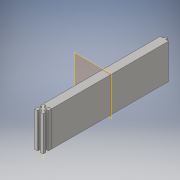
# Autodesk Inventor part: mazeblock
Saved by Autodesk Inventor 2016 (Build 200138000, 138)
## iProperties
Created: 2016-04-28
Part Number: mazeblock
Material: Generic
Document SubType Name: Modeling
Designer: brent
Density: 1 g/cm^3
Appearance: Default
Author: brent
Autodesk Inventor part; units mm, degrees
ref_plane "YZ Plane" through (0, 0, 0) normal (1, 0, 0) x (0, 1, 0)
ref_plane "XZ Plane" through (0, 0, 0) normal (0, 1, 0) x (-1, 0, 0)
ref_plane "XY Plane" through (0, 0, 0) normal (0, 0, 1) x (1, 0, 0)
sketch "Sketch1" plane through (0, 0, 0) normal (0, 1, 0) x (-1, 0, 0)
  line L0 (0, 0) -> (-180, 0) construction
  line L1 (-180, 0) -> (-180, -180) construction
  line L2 (-180, -180) -> (0, -180) construction
  line L3 (0, -180) -> (0, 0) construction
  line L4 (-6, 6) -> (6, 6)
  line L5 (6, 6) -> (6, -6)
  line L6 (6, -6) -> (1.2361, -6)
  line L7 (-6, -6) -> (-6, 6)
  line L8 (-6, 6) -> (6, -6) construction
  line L9 (6, 6) -> (-6, -6) construction
  line L10 (-6, -174) -> (6, -174)
  line L11 (6, -174) -> (6, -186)
  line L12 (6, -186) -> (-6, -186)
  line L13 (-6, -186) -> (-6, -174)
  line L14 (-6, -174) -> (6, -186) construction
  line L15 (6, -174) -> (-6, -186) construction
  line L16 (-6, -6.2) -> (6, -6.2)
  line L17 (6, -6.2) -> (6, -173.8)
  line L18 (6, -173.8) -> (-6, -173.8)
  line L19 (-6, -173.8) -> (-6, -6.2)
  line L20 (-6, -6.2) -> (6, -173.8) construction
  line L21 (6, -6.2) -> (-6, -173.8) construction
  line L22 (0, -2.1958) -> (2, -3.6489)
  line L23 (2, -3.6489) -> (1.2361, -6)
  line L24 (-1.2361, -6) -> (-2, -3.6489)
  line L25 (-2, -3.6489) -> (0, -2.1958)
  line L26 (0, -2.4739) -> (1.7355, -3.7348)
  line L27 (1.7355, -3.7348) -> (1.0726, -5.775)
  line L28 (-1.0726, -5.775) -> (-1.7355, -3.7348)
  line L29 (-1.7355, -3.7348) -> (0, -2.4739)
  line L30 (1.0726, -5.775) -> (0.9345, -6.2)
  line L31 (-1.0726, -5.775) -> (-0.9345, -6.2)
  line L32 (1.2361, -6) -> (-1.2361, -6)
  line L33 (-1.2361, -6) -> (-6, -6)
  line L34 (6, -6.2) -> (5, -6.2)
  line L35 (5, -6.2) -> (5, -6.15)
  line L36 (5, -6.15) -> (6, -6.15)
  line L37 (6, -6.15) -> (6, -6.2)
  line L38 (-5, -6.2) -> (-5, -6.15)
  line L39 (-5, -6.15) -> (-6, -6.15)
  line L40 (-6, -6.15) -> (-6, -6.2)
  line L41 (5, -6.2) -> (6, -6.2)
  line L42 (-6, -6.2) -> (-5, -6.2)
  point P0 (0, -90)
  point P1 (0, -4.2987)
  point P2 (0, -4.2987)
  dimension "d0" = 180
  dimension "d1" = 180
  dimension "d4" = 12
  dimension "d5" = 12
  dimension "d6" = 0.2
  dimension "d7" = 4
  dimension "d8" = 0.225
  dimension "d22" = 12
  dimension "d24" = 1
  dimension "d25" = 0.15
  constraints: 86 end point, 12 parallel, 7 midpoint, 7 point on line, 6 horizontal, 5 perpendicular, 3 symmetric about line, 2 collinear, 1 coincident, 18 other
  measures "d0" distance of L2.end L1.end
  measures "d1" distance of L1.end L0.end
  measures "d4" distance of L11.end L12.end
  measures "d5" distance of L10.end L11.end
  measures "d6" distance between parallel lines of L6 L16
  measures "d7" distance of L22.end L24.end
  measures "d8" distance between parallel lines of L22 L26
  measures "d22" distance of L4.end L5.end
  measures "d24" distance of L35.end L36.end
  measures "d25" distance between parallel lines of L6 L36
extrude "Extrusion1" add sketch "Sketch1" along normal blind 50 contours L4 L5 L6 L23 L22 L25 L24 L33 L7 | L24 L25 L22 L23 L32 L30 L27 L26 L29 L28 L31 | L31 L28 L29 L26 L27 L30 L32
extrude "Extrusion2" cut sketch "Sketch1" along normal through all contours L24 L25 L22 L23 L32 L30 L27 L26 L29 L28 L31 | L31 L28 L29 L26 L27 L30 L32
pattern_circular "Circular Pattern1" count 4 over 360 about axis through (0, 0, 0) along (0, -1, 0) of "Extrusion2"
extrude "Extrusion3" add sketch "Sketch1" along normal blind 50 separate body contours L16 L17 L18 L19
extrude "Extrusion4" add sketch "Sketch1" along normal up to surface (50 mm away) contours L32 L30 L16 L31 | L31 L28 L29 L26 L27 L30 L32 | L16 L40 L39 L38 | L35 L36 L37 L16 bodies 2
fillet "Fillet1" radius 0.75 8 edges at (1.2361, 25, -6) (-1.2361, 25, -6) (6, 25, -1.2361) (6, 25, 1.2361) (1.2361, 25, 6) (-6, 25, -1.2361) (-6, 25, 1.2361) (-1.2361, 25, 6)
ref_plane "Work Plane2" through (6, 0, -90) normal (0, 0, 1) x (1, 0, 0)
mirror "Mirror2" about plane through (6, 0, -90) normal (0, 0, 1) of "Extrusion4" bodies 2
fillet "Fillet3" radius 1 4 edges at (0.9345, 25, -6.2) (-0.9345, 25, -6.2) (0.9345, 25, -173.8) (-0.9345, 25, -173.8)
body "Solid1"
body "Solid2"
